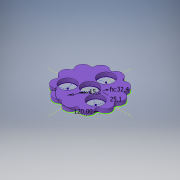
# Autodesk Inventor part: Excenter
Saved by Autodesk Inventor 2018.3 (Build 223284000, 284)
## iProperties
Created: 2018-07-20
Part Number: Excenter
Material: Generisch
Document SubType Name: Modeling
Designer: JochenAlt
Density: 1 g/cm^3
Appearance: Violett
Author: JochenAlt
Autodesk Inventor part; units mm, degrees
ref_plane "YZ Plane" through (0, 0, 0) normal (1, 0, 0) x (0, 1, 0)
ref_plane "XZ Plane" through (0, 0, 0) normal (0, 1, 0) x (-1, 0, 0)
ref_plane "XY Plane" through (0, 0, 0) normal (0, 0, 1) x (1, 0, 0)
sketch "Skizze1" plane through (0, 0, 0) normal (0, 0, 1) x (1, 0, 0)
  line L0 (0, 42.1516) -> (0, -42.1516) construction
  line L1 (-41.3732, 0) -> (41.8593, 0) construction
  circle A0 centre (0, 0) radius 7.6
  line L2 (0, 0) -> (25.1147, -14.5) construction
  line L3 (0, 0) -> (-25.1147, -14.5) construction
  circle A1 centre (14.0296, -8.1) radius 7.6
  circle A2 centre (-14.0296, -8.1) radius 7.6
  circle A3 centre (0, 16.2) radius 7.6
  circle A4 centre (0, 0) radius 16.2 construction
  spline S0 degree 5 poles (25.1, 0) (25.101, -0.5159) (25.2686, -1.1568) (25.6366, -1.5502) (26.434, -2.1028) (27.0262, -2.8656) (27.247, -3.2003) (27.7065, -4.12) (27.9538, -5.1023) (28.0285, -5.7197) (28.0371, -7.0043) (27.7442, -8.2646) (27.5105, -8.9019) (26.9448, -10.0086) (26.1342, -10.958) (25.7231, -11.3406) (24.9762, -11.8917) (24.1451, -12.2496) (23.8131, -12.3701) (22.7122, -12.5783) (21.5984, -12.6788) (20.9179, -13.484) (20.6125, -14.5462) (20.9008, -15.6782) (21.0272, -15.9695) (21.1876, -16.7843) (21.1923, -17.5737) (21.1283, -18.0572) (20.885, -19.135) (20.3879, -20.1527) (20.0375, -20.6912) (19.1952, -21.7019) (18.1448, -22.4821) (17.5668, -22.8138) (16.4794, -23.2685) (15.3228, -23.462) (14.8064, -23.4919) (13.9868, -23.4435) (13.1835, -23.2191) (12.9012, -23.1111) (11.8728, -22.581) (10.771, -22.4308) (9.7428, -22.9216) (9.2528, -23.9305) (8.9708, -25.0409) (8.8417, -25.3314) (8.456, -26.0858) (7.9033, -26.7432) (7.5214, -27.1076) (6.5612, -27.8349) (5.4654, -28.3205) (4.8197, -28.5159) (3.5351, -28.7411) (2.2278, -28.6597) (1.6024, -28.5455) (0.5568, -28.2197) (-0.3748, -27.6718) (-0.7455, -27.4033) (-1.3465, -26.8422) (-1.8282, -26.1489) (-1.9736, -25.8131) (-2.7596, -24.9414) (-3.8201, -24.638) (-4.7679, -24.7377) (-5.4828, -25.5494) (-6.3869, -26.1817) (-6.7064, -26.3539) (-7.5799, -26.7282) (-8.5151, -26.9021) (-9.1004, -26.939) (-10.3586, -26.8767) (-11.5738, -26.521) (-12.1953, -26.2538) (-13.3045, -25.605) (-14.2204, -24.727) (-14.6118, -24.2572) (-15.1351, -23.4378) (-15.4822, -22.5007) (-15.5677, -22.1393) (-15.7397, -21.0903) (-15.5675, -20.0836) (-15.8936, -19.3663) (-16.695, -18.5881) (-17.8484, -18.3465) (-18.2882, -18.4413) (-19.1542, -18.6075) (-20.0439, -18.5294) (-20.458, -18.4572) (-21.4768, -18.1536) (-22.3906, -17.6419) (-22.9012, -17.2659) (-23.8483, -16.3817) (-24.5672, -15.296) (-24.8691, -14.6897) (-25.2772, -13.5392) (-25.4096, -12.3166) (-25.4056, -11.7744) (-25.301, -10.8839) (-25.0038, -10.0657) (-24.8747, -9.7543) (-24.2576, -8.8043) (-23.6965, -7.8253) (-23.9454, -6.7418) (-24.6723, -5.9067) (-25.7445, -5.4531) (-26.0199, -5.337) (-26.724, -4.9004) (-27.3038, -4.3588) (-27.626, -3.9686) (-28.2605, -3.0245) (-28.6691, -1.9405) (-28.8221, -1.3045) (-28.9779, 0) (-28.8221, 1.3045) (-28.6691, 1.9405) (-28.2605, 3.0245) (-27.626, 3.9686) (-27.3038, 4.3588) (-26.724, 4.9004) (-26.0199, 5.337) (-25.7445, 5.4531) (-24.6723, 5.9067) (-23.9454, 6.7418) (-23.6965, 7.8253) (-24.2576, 8.8043) (-24.8747, 9.7543) (-25.0038, 10.0657) (-25.301, 10.8839) (-25.4056, 11.7744) (-25.4096, 12.3166) (-25.2772, 13.5392) (-24.8691, 14.6897) (-24.5672, 15.296) (-23.8483, 16.3817) (-22.9012, 17.2659) (-22.3906, 17.6419) (-21.4768, 18.1536) (-20.458, 18.4572) (-20.0439, 18.5294) (-19.1542, 18.6075) (-18.2882, 18.4413) (-17.8484, 18.3465) (-16.695, 18.5881) (-15.8936, 19.3663) (-15.5675, 20.0836) (-15.7397, 21.0903) (-15.5677, 22.1393) (-15.4822, 22.5007) (-15.1351, 23.4378) (-14.6118, 24.2572) (-14.2204, 24.727) (-13.3045, 25.605) (-12.1953, 26.2538) (-11.5738, 26.521) (-10.3586, 26.8767) (-9.1004, 26.939) (-8.5151, 26.9021) (-7.5799, 26.7282) (-6.7064, 26.3539) (-6.3869, 26.1817) (-5.4828, 25.5494) (-4.7679, 24.7377) (-3.8201, 24.638) (-2.7596, 24.9414) (-1.9736, 25.8131) (-1.8282, 26.1489) (-1.3465, 26.8422) (-0.7455, 27.4033) (-0.3748, 27.6718) (0.5568, 28.2197) (1.6024, 28.5455) (2.2278, 28.6597) (3.5351, 28.7411) (4.8197, 28.5159) (5.4654, 28.3205) (6.5612, 27.8349) (7.5214, 27.1076) (7.9033, 26.7432) (8.456, 26.0858) (8.8417, 25.3314) (8.9708, 25.0409) (9.2528, 23.9305) (9.7428, 22.9216) (10.771, 22.4308) (11.8728, 22.581) (12.9012, 23.1111) (13.1835, 23.2191) (13.9868, 23.4435) (14.8064, 23.4919) (15.3228, 23.462) (16.4794, 23.2685) (17.5668, 22.8138) (18.1448, 22.4821) (19.1952, 21.7019) (20.0375, 20.6912) (20.3879, 20.1527) (20.885, 19.135) (21.1283, 18.0572) (21.1923, 17.5737) (21.1876, 16.7843) (21.0272, 15.9695) (20.9008, 15.6782) (20.6125, 14.5462) (20.9179, 13.484) (21.5984, 12.6788) (22.7122, 12.5783) (23.8131, 12.3701) (24.1451, 12.2496) (24.9762, 11.8917) (25.7231, 11.3406) (26.1342, 10.958) (26.9448, 10.0086) (27.5105, 8.9019) (27.7442, 8.2646) (28.0371, 7.0043) (28.0285, 5.7197) (27.9538, 5.1023) (27.7065, 4.12) (27.247, 3.2003) (27.0262, 2.8656) (26.434, 2.1028) (25.6366, 1.5502) (25.2686, 1.1568) (25.101, 0.5159) (25.1, 0) knots 0 0 0 0 0 0 0.013794 0.013794 0.013794 0.023969 0.023969 0.023969 0.03927 0.03927 0.03927 0.05615 0.05615 0.05615 0.070317 0.070317 0.070317 0.079 0.079 0.079 0.098426 0.098426 0.098426 0.106883 0.106883 0.106883 0.118655 0.118655 0.118655 0.134809 0.134809 0.134809 0.151359 0.151359 0.151359 0.16415 0.16415 0.16415 0.171997 0.171997 0.171997 0.192425 0.192425 0.192425 0.200409 0.200409 0.200409 0.213683 0.213683 0.213683 0.230379 0.230379 0.230379 0.246282 0.246282 0.246282 0.257526 0.257526 0.257526 0.267053 0.267053 0.267053 0.285251 0.285251 0.285251 0.294398 0.294398 0.294398 0.308971 0.308971 0.308971 0.325888 0.325888 0.325888 0.340839 0.340839 0.340839 0.35049 0.35049 0.35049 0.36678 0.36678 0.36678 0.378112 0.378112 0.378112 0.388823 0.388823 0.388823 0.40444 0.40444 0.40444 0.421246 0.421246 0.421246 0.43498 0.43498 0.43498 0.443264 0.443264 0.443264 0.463382 0.463382 0.463382 0.471341 0.471341 0.471341 0.48363 0.48363 0.48363 0.5 0.5 0.5 0.51637 0.51637 0.51637 0.528659 0.528659 0.528659 0.536618 0.536618 0.536618 0.556736 0.556736 0.556736 0.56502 0.56502 0.56502 0.578754 0.578754 0.578754 0.59556 0.59556 0.59556 0.611177 0.611177 0.611177 0.621888 0.621888 0.621888 0.63322 0.63322 0.63322 0.64951 0.64951 0.64951 0.659161 0.659161 0.659161 0.674112 0.674112 0.674112 0.691029 0.691029 0.691029 0.705602 0.705602 0.705602 0.714749 0.714749 0.714749 0.732947 0.732947 0.732947 0.742474 0.742474 0.742474 0.753718 0.753718 0.753718 0.769621 0.769621 0.769621 0.786317 0.786317 0.786317 0.799591 0.799591 0.799591 0.807575 0.807575 0.807575 0.828003 0.828003 0.828003 0.83585 0.83585 0.83585 0.848641 0.848641 0.848641 0.865191 0.865191 0.865191 0.881345 0.881345 0.881345 0.893117 0.893117 0.893117 0.901574 0.901574 0.901574 0.921 0.921 0.921 0.929683 0.929683 0.929683 0.94385 0.94385 0.94385 0.96073 0.96073 0.96073 0.976031 0.976031 0.976031 0.986206 0.986206 0.986206 1 1 1 1 1 1
  circle A5 centre (0, 0) radius 25.1 construction
  dimension "d1" = 15.2
  dimension "d2" = 120
  dimension "d3" = 32.4
  dimension "d12" = 25.1
  constraints: 5 centre point, 4 end point, 4 point on line, 3 equal radius, 3 point on circle, 2 coincident, 1 horizontal alignment, 5 other
  measures "d1" diameter of A0
  measures "d2" angle of L2 L3
  measures "d3" diameter of A4
  measures "d12" distance of point (25.1, 0) L2.start
extrude "Extrusion1" add sketch "Skizze1" along normal blind 4
equation "curve S0 of \"Skizze1\": x = (29*cos(t))-(2*cos(t+atan(sin(-11*t)/((29/1,9/12)-cos(-11*t)))))-(1,9*cos(12*t)); y = (-29*sin(t))+(2*sin(t+atan(sin(-11*t)/((29/1,9/12)-cos(-11*t)))))+(1,9*sin(12*t)); t fr"
